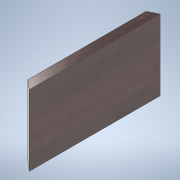
# Autodesk Inventor part: WinchWall-ver1-1111-2021
Saved by Autodesk Inventor 2021 (Build 250183000, 183)
## iProperties
Created: 2021-03-03
Part Number: WinchWall-ver1-1111-2021
Material: Generic
Document SubType Name: Modeling
Designer: CMurray
Density: 1 g/cm^3
Appearance: Wild Cherry - Wild Berries
Author: CMurray
Autodesk Inventor part; units mm, degrees
ref_plane "YZ Plane" through (0, 0, 0) normal (1, 0, 0) x (0, 1, 0)
ref_plane "XZ Plane" through (0, 0, 0) normal (0, 1, 0) x (-1, 0, 0)
ref_plane "XY Plane" through (0, 0, 0) normal (0, 0, 1) x (1, 0, 0)
sketch "Sketch2" plane through (0, 0, 0) normal (0, 1, 0) x (-1, 0, 0)
  line L0 (429.133, -156.7133) -> (429.133, -791.7227)
  line L1 (378.333, -113.257) -> (378.333, -817.2173)
  arc A0 (378.333, -817.2173) -> (429.133, -791.7227) centre (0, 0) ccw
  line L2 (429.133, -156.7133) -> (378.333, -113.257)
  point P0 (429.133, 791.7227)
  constraints: 6 end point, 2 point on circle, 1 centre point, 1 coincident, 1 point on line, 1 vertical
extrude "Extrusion2" add sketch "Sketch2" along normal blind 381
body "Solid2"
